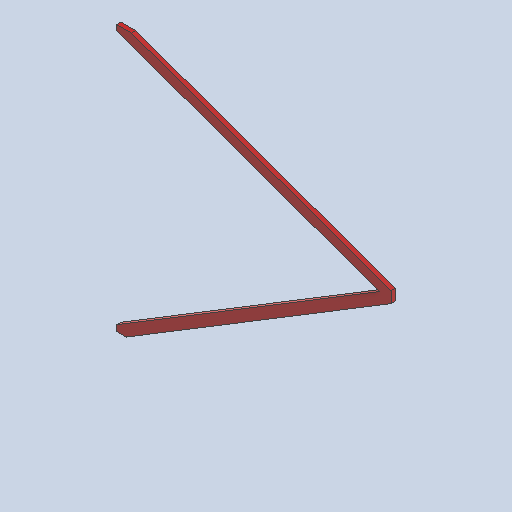
# Autodesk Inventor part: s58x2x4
Saved by Autodesk Inventor 2025.1 (Build 291241020, 241B)
## iProperties
Created: 2024-09-16
Part Number: s58x2x4
Material: Generic
Document SubType Name: Modeling
Designer: User
Density: 1 g/cm^3
Appearance: Default
Stock Number: 2x10
Author: User
Autodesk Inventor part; units mm, degrees
ref_plane "YZ Plane" through (0, 0, 0) normal (1, 0, 0) x (0, 1, 0)
ref_plane "XZ Plane" through (0, 0, 0) normal (0, 1, 0) x (-1, 0, 0)
ref_plane "XY Plane" through (0, 0, 0) normal (0, 0, 1) x (1, 0, 0)
sketch "Sketch1" plane through (0, 0, 0) normal (0, 0, 1) x (1, 0, 0)
  line L0 (-2438.4, -2400.3) -> (0, -2400.3) projected
  line L1 (0, -2438.4) -> (0, 2438.4) projected
  line L2 (0, -38.1) -> (-2438.4, -38.1) projected
  line L3 (-2438.4, 1219.2) -> (-2438.4, -2438.4) projected
  line L4 (-2438.4, -2348.2472) -> (-102.4888, -924.8013)
  line L5 (-102.4888, -924.8013) -> (-2438.4, -85.3332)
  line L6 (-2306.9684, -38.1) -> (0, -867.1668)
  line L7 (0, -966.4528) -> (-2352.98, -2400.3)
  line L8 (0, -867.1668) -> (0, -966.4528)
  line L9 (-2352.98, -2400.3) -> (-2438.4, -2400.3)
  line L10 (-2438.4, -2400.3) -> (-2438.4, -2348.2472)
  line L11 (-2438.4, -85.3332) -> (-2438.4, -38.1)
  line L12 (-2438.4, -38.1) -> (-2306.9684, -38.1)
  point P0 (0, 0)
  constraints: 18 end point, 6 point on line, 5 collinear, 2 parallel, 4 other
extrude "Extrusion1" add sketch "Sketch1" against normal blind 38.1 contours L3 L4 L5 L2 L6 L1 L7 L0
body "Solid1"
